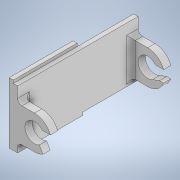
# Autodesk Inventor part: Lid
Saved by Autodesk Inventor 2020 (Build 240168000, 168)
## iProperties
Created: 2019-09-30
Part Number: Lid
Material: Generic
Document SubType Name: Modeling
Designer: bzs3334
Density: 1 g/cm^3
Appearance: Default
Mass: 21.9269 g
Surface Area: 97.0217 cm^2
Volume: 21.9269 cm^3
Author: bzs3334
Autodesk Inventor part; units mm, degrees
ref_plane "YZ Plane" through (0, 0, 0) normal (1, 0, 0) x (0, 1, 0)
ref_plane "XZ Plane" through (0, 0, 0) normal (0, 1, 0) x (-1, 0, 0)
ref_plane "XY Plane" through (0, 0, 0) normal (0, 0, 1) x (1, 0, 0)
sketch "Sketch1" plane through (0, 0, 0) normal (1, 0, 0) x (0, 1, 0)
  line L0 (21, 41.5) -> (-21, 41.5)
  line L1 (-21, 41.5) -> (-21, -41.5)
  line L2 (-21, -41.5) -> (21, -41.5)
  line L3 (21, -41.5) -> (21, 41.5)
  point P0 (0, 0)
  dimension "d0" = 83
  dimension "d1" = 41.5
  dimension "d2" = 42
  dimension "d3" = 21
  constraints: 8 end point, 2 parallel, 1 horizontal, 1 perpendicular
  measures "d0" distance of L2.end L0.start
  measures "d1" distance from line of L0 point (0, 0)
  measures "d2" distance of L0.start L0.end
  measures "d3" horizontal distance of L0.end point (0, 0)
extrude "Extrusion1" add sketch "Sketch1" along normal blind 2.85
sketch "Sketch3" plane through (2.85, 0, 0) normal (1, 0, 0) x (0, 0, -1)
  line L0 (41.5, 21) -> (-41.5, 21) projected
  line L1 (-41.5, 21) -> (2.5, 21)
  line L2 (2.5, 21) -> (2.5, 19)
  line L3 (2.5, 19) -> (-41.5, 19)
  line L4 (-41.5, 19) -> (-41.5, 21)
  line L5 (-41.5, -21) -> (41.5, -21) projected
  line L6 (41.5, -21) -> (3.5, -21)
  line L7 (3.5, -21) -> (3.5, -19)
  line L8 (3.5, -19) -> (41.5, -19)
  line L9 (41.5, -19) -> (41.5, -21)
  line L10 (41.5, -21) -> (41.5, 21) projected
  line L11 (41.5, 21) -> (-41.5, 21) projected
  line L12 (-41.5, 21) -> (-41.5, -21) projected
  line L13 (-41.5, -21) -> (41.5, -21) projected
  point P0 (0, 0)
  point P1 (41.5, 21)
  dimension "d12" = 44
  dimension "d13" = 2
  dimension "d14" = 38
  dimension "d15" = 2
  constraints: 16 end point, 4 parallel, 2 horizontal, 2 perpendicular
  measures "d12" distance of L2.end L3.end
  measures "d13" distance of L1.end L2.end
  measures "d14" distance of L7.end L8.end
  measures "d15" distance of L6.end L7.end
extrude "Extrusion3" add sketch "Sketch3" along normal blind 3 contours L10 L8 L7 L5 L12 L3 L2 L0
sketch "Sketch4" plane through (0, 21, 41.5) normal (0, 1, 0) x (1, 0, 0)
  line L0 (0, 83) -> (0, 0) projected
  line L1 (2.85, 44) -> (5.85, 44) projected
  line L2 (0, 83) -> (5.85, 83)
  line L3 (5.85, 83) -> (5.85, 44)
  line L4 (5.85, 44) -> (0, 44)
  line L5 (0, 44) -> (0, 83)
  point P0 (0, 41.5)
  constraints: 8 end point, 2 parallel, 1 horizontal, 1 perpendicular
extrude "Extrusion4" cut sketch "Sketch4" against normal blind 6.5
sketch "Sketch5" plane through (0, -21, 41.5) normal (0, 0, 1) x (1, 0, 0)
  circle A0 centre (17.475, 18) radius 6.625
  circle A1 centre (17.475, 18) radius 11.625
  line L0 (5.85, 40) -> (5.85, 0) projected
  line L1 (5.85, 2) -> (5.85, 35.5) projected
  line L2 (2.85, 40) -> (5.85, 40) projected
  line L3 (17.475, 6.375) -> (5.85, 6.375)
  line L4 (28.3902, 22) -> (12.1938, 22)
  line L5 (28.3902, 14) -> (12.1938, 14)
  line L6 (17.475, 29.625) -> (5.85, 29.625)
  line L7 (17.475, 18) -> (5.85, 18)
  line L8 (0, 0) -> (5.85, 0) projected
  point P0 (0, 21)
  point P1 (22.7562, 14)
  point P2 (22.7562, 22)
  dimension "d20" = 13.25
  dimension "d21" = 5
  dimension "d30" = 18
  dimension "d31" = 4
  dimension "d32" = 4
  constraints: 10 end point, 7 point on circle, 3 perpendicular, 3 point on line, 3 tangent, 2 centre point, 1 horizontal, 1 parallel
  measures "d20" diameter of A0
  measures "d21" radial gap between concentric circles of A0 A1
  measures "d30" distance between parallel lines of L8 L7
  measures "d31" distance between parallel lines of L4 L7
  measures "d32" distance between parallel lines of L5 L7
extrude "Extrusion5" add sketch "Sketch5" against normal blind 5 contours A0 L7 A1 L4 | L5 A1 L7 A0 | A1 L0 L6 | L3 L0 A1
fillet "Fillet3" radius 3 3 edges at (5.85, -14.625, 39) (5.85, -3, 36.5) (5.85, 8.625, 39)
ref_plane "Work Plane1" through (2.85, -21, 0) normal (0, 0, -1) x (-1, 0, 0)
mirror "Mirror1" about plane through (2.85, -21, 0) normal (0, 0, -1) of "Extrusion5", "Fillet3"
sketch "Sketch6" plane through (0, -21, 36.5) normal (0, 0, -1) x (-1, 0, 0)
  line L0 (-8.85, 29.625) -> (-8.85, 6.375) projected
  line L1 (-8.85, 29.625) -> (-17.475, 29.625) projected
  arc A0 (-17.475, 29.625) -> (-28.3902, 22) centre (-17.475, 18) ccw projected
  line L2 (-28.3902, 22) -> (-22.7562, 22) projected
  arc A1 (-22.7562, 14) -> (-22.7562, 22) centre (-17.475, 18) ccw projected
  line L3 (-22.7562, 14) -> (-28.3902, 14) projected
  arc A2 (-28.3902, 14) -> (-17.475, 6.375) centre (-17.475, 18) ccw projected
  line L4 (-17.475, 6.375) -> (-8.85, 6.375) projected
  line L5 (-17.475, 18) -> (-23.2875, 28.0675)
  arc A3 (-17.475, 29.625) -> (-28.3902, 22) centre (-17.475, 18) ccw projected
  line L6 (-17.475, 18) -> (-5.85, 18) construction
  line L7 (-17.475, 18) -> (-23.2875, 7.9325)
  arc A4 (-28.3902, 14) -> (-17.475, 6.375) centre (-17.475, 18) ccw projected
  line L8 (-17.475, 18) -> (-5.85, 18) construction
  point P0 (0, 21)
  point P1 (-20.7875, 23.7374)
  point P2 (-20.7875, 12.2626)
  dimension "d33" = 120
  dimension "d42" = 120
  constraints: 8 end point, 2 equal length, 2 horizontal, 2 point on circle
  measures "d33" angle of L6 L5
  measures "d42" angle of L7 L8
extrude "Extrusion6" cut sketch "Sketch6" against normal blind 13.5 contours A2 L3 A1 L7
sketch "Sketch7" plane through (2.85, -21, -41.5) normal (0, 0, -1) x (-1, 0, 0)
  line L0 (2.85, 35.5) -> (-3, 35.5) projected
  line L1 (-3, 32.625) -> (-3, 35.5) projected
  arc A0 (-6, 29.625) -> (-3, 32.625) centre (-6, 32.625) ccw projected
  line L2 (-14.625, 29.625) -> (-6, 29.625) projected
  arc A1 (-14.625, 29.625) -> (-25.5402, 22) centre (-14.625, 18) ccw projected
  line L3 (-19.9062, 22) -> (-25.5402, 22) projected
  arc A2 (-19.9062, 14) -> (-19.9062, 22) centre (-14.625, 18) ccw projected
  line L4 (-25.5402, 14) -> (-19.9062, 14) projected
  arc A3 (-25.5402, 14) -> (-14.625, 6.375) centre (-14.625, 18) ccw projected
  line L5 (-6, 6.375) -> (-14.625, 6.375) projected
  arc A4 (-3, 3.375) -> (-6, 6.375) centre (-6, 3.375) ccw projected
  line L6 (-3, 2) -> (-3, 3.375) projected
  line L7 (0, 2) -> (-3, 2) projected
  line L8 (0, 0) -> (0, 2) projected
  line L9 (2.85, 0) -> (0, 0) projected
  line L10 (2.85, 0) -> (2.85, 35.5) projected
  arc A5 (-14.625, 29.625) -> (-25.5402, 22) centre (-14.625, 18) ccw projected
  line L11 (-19.9062, 22) -> (-25.5402, 22) projected
  line L12 (-14.625, 18) -> (-20.4375, 7.9325)
  arc A6 (-25.5402, 14) -> (-14.625, 6.375) centre (-14.625, 18) ccw projected
  line L13 (-14.625, 18) -> (-3, 18) construction
  line L14 (-25.5402, 14) -> (-19.9062, 14) projected
  arc A7 (-19.9062, 14) -> (-19.9062, 22) centre (-14.625, 18) ccw projected
  line L15 (-17.9375, 12.2626) -> (-22.711, 14)
  line L16 (-17.9375, 12.2626) -> (-12.8576, 12.2626) construction
  point P0 (2.85, 21)
  dimension "d43" = 120
  dimension "d44" = 160
  constraints: 8 end point, 2 equal length, 2 horizontal, 1 point on circle, 1 point on line
  measures "d43" angle of L12 L13
  measures "d44" angle of L16 L15
extrude "Extrusion7" cut sketch "Sketch7" against normal blind 11.5 contours L15 L4 A2
sketch "Sketch8" plane through (0, 14.5, 41.5) normal (0, 1, 0) x (1, 0, 0)
  line L0 (2.85, 44) -> (0, 44) projected
  line L1 (0, 83) -> (5.85, 83) projected
  line L2 (2.85, 44) -> (5.85, 44)
  line L3 (5.85, 44) -> (5.85, 83)
  line L4 (5.85, 83) -> (2.85, 83)
  line L5 (2.85, 83) -> (2.85, 44)
  point P0 (0, 41.5)
  constraints: 8 end point, 2 parallel, 1 horizontal, 1 perpendicular
extrude "Extrusion8" add sketch "Sketch8" along normal up to surface (4.5 mm away)
equation "\"d1\" = 0.5 * d0"
equation "\"d3\" = 0.5 * d2"
equation "\"d32\" = d31"
body "Solid1"
